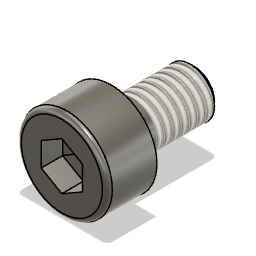
fusion_export (Autodesk Fusion 360 archive; units mm, degrees)
design "Innensechskantschraube DIN EN ISO 4762 - M3 x 5 Stahl 4.6 Einfach"
description: Innensechskantschraube DIN EN ISO 4762 - M3 x 5
Autodesk Fusion 360 part; units mm, degrees
note: some values were not read from the file. Chosen so that the rebuilt part matches the saved one: how an offset face is resized. Set by a fixed rule: which sketch regions a step uses.
sketch "Sketch1" plane through (0, 0, 0) normal (0, 1, 0) x (1, 0, 0)
  line L0 (-1.5, 0) -> (-1.5, 5)
  line L1 (-1.5, 5) -> (0, 5)
  line L2 (0, 5) -> (0, -3)
  line L3 (-1.5, 0) -> (-2.75, 0)
  line L4 (-2.75, 0) -> (-2.75, -3)
  line L5 (-2.75, -3) -> (0, -3)
  dimension "d9" = 3
  dimension "d66" = 5.5
  dimension "d68" = 5
  dimension "d79" = 3
  constraint perpendicular L0 L1
  constraint collinear origin L1.end L2.end
  constraint perpendicular L0 L3
  constraint coincident origin L3
  constraint vertical L0
  constraint vertical L2
  constraint parallel L2 L4
  constraint coincident L2 L5.end
  constraint perpendicular L2 L5
  measures "d68" distance of origin L1.end
  measures "d79" distance of L3.end L4.end
revolve "Revolve1" add sketch "Sketch1" angle 360 about axis through (0, 0, -5) along (0, 0, 1)
ref_plane "WorkPlane1" through (0, 0, 3) normal (0, 0, 1) x (1, 0, 0)
sketch "Sketch6" plane through (0, 0, 3) normal (0, 0, 1) x (1, 0, 0)
  line L0 (-1.25, 0) -> (1.25, 0) construction
  line L1 (0, 0) -> (-1.25, 0.7217)
  line L2 (-1.25, -0.7217) -> (-1.25, 0.7217)
  line L3 (-1.25, -0.7217) -> (0, 0)
  dimension "d72" = 2.5
  dimension "d104" = 150
  constraint horizontal L0
  constraint midpoint L1.start L0
  constraint coincident L1.start L3.end
  constraint perpendicular L0 L2
  constraint midpoint L0.start L2
  constraint coincident L1.end L2.end
  measures "d72" distance of L0.start L0.end
  measures "d104" angle of L0 L1
extrude "Extrude1" cut sketch "Sketch6" against normal blind 1.3
pattern_circular "C-Pattern1" count 6 over 360 about axis through (0, 0, 1.75) along (0, 0, 1) of "Extrude1"
extrude "Extrude2" cut 1 faces at (0, -0.4811, 1.7) along direction (0, 0, -1) blind 1.3 draft -85
fillet "Fillet4" radius 0.3 1 edges at (-2.5639, 0.9944, 3)
thread "Thread2" "ISO Metric profile 3.0 M3x0.5 6g" major diameter 2.927 minor diameter 2.3555 pitch 0.5 angle 60 resizes the face on face at (-1.4925, 0.1494, -3.3333)
sketch "Sketch7" plane through (0, 0, 0) normal (0, 1, 0) x (1, 0, 0)
  line L0 (-1.53, 5) -> (-1.53, 4.7)
  line L1 (-1.53, 4.7) -> (-1.23, 5)
  line L2 (0, 5) -> (0, -3)
  line L3 (-1.53, 5) -> (0, 5)
  dimension "d99" = 1.53
  dimension "d101" = 45
  dimension "d103" = 0.3
  constraint coincident L2.start L3.end
  constraint perpendicular L2 L3
  constraint coincident L1.end L3
  constraint perpendicular L0 L3
  measures "d99" distance of origin L0
  measures "d101" angle of L0 L1
  measures "d103" vertical distance of L0.end L1.end
revolve "Revolve3" cut sketch "Sketch7" angle 360 about axis through (0, 0, 1.75) along (0, 0, 1)
equation "d9 = adsk_nomdia"
equation "adsk_nomlen = 5.00 mm"
equation "adsk_headh = 3.00 mm"
equation "adsk_headdia = 5.50 mm"
equation "adsk_nomdia = 3.00 mm"
equation "adsk_philwidth = 2.50 mm"
equation "d31 = -adsk_phildepth"
equation "adsk_phildepth = 1.30 mm"
equation "d66 = adsk_headdia"
equation "d68 = adsk_nomlen"
equation "d71 = adsk_headh"
equation "d72 = adsk_philwidth"
equation "d76 = -adsk_phildepth"
equation "d79 = adsk_headh"
equation "adsk_thrlen = 3.75 mm"
equation "d84 = adsk_thrlen"
equation "d86 = adsk_nomdia * 0.1"
equation "d99 = adsk_nomdia * 0.51"
equation "adsk_startang = 45.00 deg"
equation "d101 = adsk_startang"
equation "adsk_pitch1 = 0.50 mm"
equation "d103 = adsk_startlen"
equation "adsk_startlen = 0.30 mm"

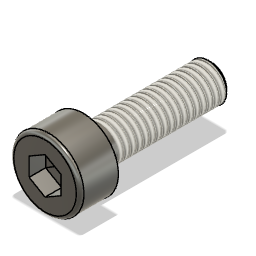
design "Innensechskantschraube DIN EN ISO 4762 - M3 x 10 Stahl 4.6 Einfach"
description: Innensechskantschraube DIN EN ISO 4762 - M3 x 10
Autodesk Fusion 360 part; units mm, degrees
sketch "Sketch1" plane through (0, 0, 0) normal (0, 1, 0) x (1, 0, 0)
  line L0 (-1.5, 0) -> (-1.5, 10)
  line L1 (-1.5, 10) -> (0, 10)
  line L2 (0, 10) -> (0, -3)
  line L3 (-1.5, 0) -> (-2.75, 0)
  line L4 (-2.75, 0) -> (-2.75, -3)
  line L5 (-2.75, -3) -> (0, -3)
  dimension "d9" = 3
  dimension "d66" = 5.5
  dimension "d68" = 10
  dimension "d79" = 3
  constraint perpendicular L0 L1
  constraint collinear origin L1.end L2.end
  constraint perpendicular L0 L3
  constraint coincident origin L3
  constraint vertical L0
  constraint vertical L2
  constraint parallel L2 L4
  constraint coincident L2 L5.end
  constraint perpendicular L2 L5
  measures "d68" distance of origin L1.end
  measures "d79" distance of L3.end L4.end
revolve "Revolve1" add sketch "Sketch1" angle 360 about axis through (0, 0, -10) along (0, 0, 1)
ref_plane "WorkPlane1" through (0, 0, 3) normal (0, 0, 1) x (1, 0, 0)
sketch "Sketch6" plane through (0, 0, 3) normal (0, 0, 1) x (1, 0, 0)
  line L0 (-1.25, 0) -> (1.25, 0) construction
  line L1 (0, 0) -> (-1.25, 0.7217)
  line L2 (-1.25, -0.7217) -> (-1.25, 0.7217)
  line L3 (-1.25, -0.7217) -> (0, 0)
  dimension "d72" = 2.5
  dimension "d104" = 150
  constraint horizontal L0
  constraint midpoint L1.start L0
  constraint coincident L1.start L3.end
  constraint perpendicular L0 L2
  constraint midpoint L0.start L2
  constraint coincident L1.end L2.end
  measures "d72" distance of L0.start L0.end
  measures "d104" angle of L0 L1
extrude "Extrude1" cut sketch "Sketch6" against normal blind 1.3
pattern_circular "C-Pattern1" count 6 over 360 about axis through (0, 0, 1.75) along (0, 0, 1) of "Extrude1"
extrude "Extrude2" cut 1 faces at (0, -0.4811, 1.7) along direction (0, 0, -1) blind 1.3 draft -85
fillet "Fillet4" radius 0.3 1 edges at (-2.5639, 0.9944, 3)
thread "Thread2" "ISO Metric profile 3.0 M3x0.5 6g" major diameter 2.927 minor diameter 2.3555 pitch 0.5 angle 60 resizes the face on face at (-1.4981, 0.0748, -3.3333)
sketch "Sketch7" plane through (0, 0, 0) normal (0, 1, 0) x (1, 0, 0)
  line L0 (-1.53, 10) -> (-1.53, 9.7)
  line L1 (-1.53, 9.7) -> (-1.23, 10)
  line L2 (0, 10) -> (0, -3)
  line L3 (-1.53, 10) -> (0, 10)
  dimension "d99" = 1.53
  dimension "d101" = 45
  dimension "d103" = 0.3
  constraint coincident L2.start L3.end
  constraint perpendicular L2 L3
  constraint coincident L1.end L3
  constraint perpendicular L0 L3
  measures "d99" distance of origin L0
  measures "d101" angle of L0 L1
  measures "d103" vertical distance of L0.end L1.end
revolve "Revolve3" cut sketch "Sketch7" angle 360 about axis through (0, 0, 1.75) along (0, 0, 1)
equation "d9 = adsk_nomdia"
equation "adsk_nomlen = 10.00 mm"
equation "adsk_headh = 3.00 mm"
equation "adsk_headdia = 5.50 mm"
equation "adsk_nomdia = 3.00 mm"
equation "adsk_philwidth = 2.50 mm"
equation "d31 = -adsk_phildepth"
equation "adsk_phildepth = 1.30 mm"
equation "d66 = adsk_headdia"
equation "d68 = adsk_nomlen"
equation "d71 = adsk_headh"
equation "d72 = adsk_philwidth"
equation "d76 = -adsk_phildepth"
equation "d79 = adsk_headh"
equation "adsk_thrlen = 8.75 mm"
equation "d84 = adsk_thrlen"
equation "d86 = adsk_nomdia * 0.1"
equation "d99 = adsk_nomdia * 0.51"
equation "adsk_startang = 45.00 deg"
equation "d101 = adsk_startang"
equation "adsk_pitch1 = 0.50 mm"
equation "d103 = adsk_startlen"
equation "adsk_startlen = 0.30 mm"
